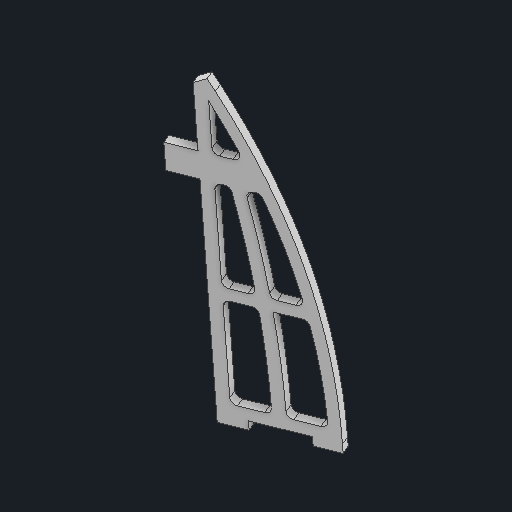
# Autodesk Inventor part: sponson_spanner_bottom
Saved by Autodesk Inventor 2023 (Build 270158030, 158C)
## iProperties
Created: 2022-03-22
Part Number: sponson_spanner_bottom
Material: Generic
Document SubType Name: Modeling
Designer: kardo
Density: 1 g/cm^3
Appearance: Default
Mass: 4.88193 g
Surface Area: 52.3251 cm^2
Volume: 4.88193 cm^3
Author: kardo
Autodesk Inventor part; units mm, degrees
ref_plane "YZ Plane" through (0, 0, 0) normal (1, 0, 0) x (0, 1, 0)
ref_plane "XZ Plane" through (0, 0, 0) normal (0, 1, 0) x (-1, 0, 0)
ref_plane "XY Plane" through (0, 0, 0) normal (0, 0, 1) x (1, 0, 0)
derived "parameters_frame.ipt"
derived "stencil_frame.ipt"
sketch "sk_joint_locations" plane through (81.12, 0, 0) normal (1, 0, 0) x (0, 1, 0)
  line L0 (0, 0) -> (122.4, 9.6331) construction
  line L1 (36.465, 28.832) -> (112.2, 28.832) construction
  arc A0 (36.465, 28.832) -> (11.22, 28.376) centre (36.465, -670.197) ccw construction
  line L2 (-241.5001, 19.2432) -> (11.22, 28.376) construction
  line L3 (-345, 16.32) -> (-262.2001, 18.586) construction
  arc A1 (-262.2001, 18.586) -> (-241.5001, 19.2432) centre (-326.8578, 2381.2399) ccw construction
  line L4 (-122.4795, 3121.122) -> (270.8781, -1876.9598) construction
  line L5 (-230.0001, 3089.1136) -> (-230.0001, -1866.0023) construction
  line L6 (-114.9999, 3089.1136) -> (-114.9999, -1866.0023) construction
  line L7 (-345, 3089.1136) -> (-345, -1866.0023) construction
  line L8 (0, 3089.1136) -> (0, -1866.0023) construction
  line L9 (529.622, 47.2379) -> (-602.608, 2.7525) construction
  line L10 (-673.1615, -36.5999) -> (647.9226, 67.3717) construction
  line L11 (189.4528, 29.5173) -> (189.1111, 38.2146) construction
  line L12 (201.105, 36.5853) -> (201.7901, 27.8813) construction
  line L13 (0, 14.144) -> (121.9006, 15.9783) construction
  line L14 (-230.0001, 45.8224) -> (-230.0001, 19.6588) construction
  line L15 (-345, 37.3935) -> (-345, 16.32) construction
  line L16 (-114.9999, 50.9907) -> (-114.9999, 23.8147) construction
  line L17 (0, 52.89) -> (0, 27.9705) construction
  line L18 (119.1768, 50.5875) -> (119.7216, 43.6656) construction
  line L19 (120.2663, 36.7438) -> (119.7216, 43.6656) construction
  line L20 (120.2663, 36.7438) -> (120.8111, 29.822) construction
  line L21 (120.8111, 29.822) -> (121.3559, 22.9001) construction
  line L22 (121.3559, 22.9001) -> (121.9006, 15.9783) construction
  line L23 (0, 14.144) -> (0, 0) construction
  line L24 (112.2, 37.536) -> (112.2, 28.832) construction
  line L25 (112.2, 35.848) -> (112.2, 30.52) construction
  spline S0 degree 4 poles (-345, 37.3935) (-258.8686, 45.1235) (-172.5923, 49.7074) (-86.3167, 52.89) (0, 52.89) knots 0 0 0 0 0 1 1 1 1 1
  spline S1 degree 3 poles (0, 52.89) (92.8353, 52.89) (195.0311, 49.5089) (255, 36.448) knots 0 0 0 0 1 1 1 1
  spline S2 degree 2 poles (122.4, 9.6331) (190.08, 14.9596) (255, 36.448) knots 0 0 0 1 1 1
  point P0 (-122.4795, 3121.122)
  point P1 (270.8781, -1876.9598)
  point P2 (189.282, 33.8659)
  point P3 (201.4475, 32.2333)
  point P4 (134.9575, 11.3411)
  point P5 (-345, 26.8568)
  point P6 (-230.0001, 32.7406)
  point P7 (-114.9999, 37.4027)
  point P8 (0, 40.4303)
  point P9 (112.2, 33.184)
sketch "sk_spanner_joints_locations" plane through (0, 122.4, 9.6331) normal (0, 0.9969173, 0.0784591) x (-1, 0, 0)
  line L0 (328.7115, -3.4565) -> (-466.2934, 45.1587) construction
  line L1 (-867.9776, -269.6459) -> (1175.5999, 473.0692) construction
  line L2 (-94.4551, 22.4205) -> (-92.9508, 12.0288) construction
  line L3 (-94.4551, 22.4205) -> (-68.6928, 20.8451) construction
  line L4 (-92.9508, 12.0288) -> (-68.6928, 20.8451) construction
  point P0 (0, 0)
  point P1 (-126.048, 0)
  point P2 (-156, 26.184)
  point P3 (-143.691, 25.4313)
  point P4 (-106.7641, 23.1732)
  point P5 (-101.2251, 9.0216)
  point P6 (-117.7737, 3.0072)
ref_plane "plane_strnger_outer" through (84.12, 0, 0) normal (1, 0, 0) x (0, 1, 0)
sketch "sk_corner_offset" plane through (0, 122.4, 9.6331) normal (0, 0.9969173, 0.0784591) x (-1, 0, 0)
  line L0 (-156, 26.184) -> (-126.048, 0) construction
  line L1 (-126.048, 0) -> (-81.12, 0) construction
  point P0 (0, 0)
  point P1 (-125.7476, 0.8)
  dimension "d7" = 0.8
  dimension "d8" = 0.8
  constraints: 4 end point, 1 horizontal
  measures "d7" distance from line of L0 point (-125.748, 0.8)
  measures "d8" distance from line of point (-125.748, 0.8) L1
sketch "sk_tip_offset" plane through (81.12, 0, 0) normal (1, 0, 0) x (0, 1, 0)
  spline S0 degree 3 poles (0, 52.89) (92.8353, 52.89) (195.0311, 49.5089) (255, 36.448) knots 0 0 0 0 1 1 1 1 construction
  spline S1 degree 2 poles (122.4, 9.6331) (190.08, 14.9596) (255, 36.448) knots 0 0 0 1 1 1 construction
  spline S2 degree 5 poles (0, 52.09) (14.1126, 52.09) (28.2252, 52.0249) (42.3374, 51.8877) (70.3021, 51.4557) (98.2587, 50.655) (112.105, 50.1551) (138.5853, 48.9703) (165.0353, 47.2425) (177.6496, 46.2711) (200.1482, 44.2213) (222.5619, 41.3963) (232.3977, 39.9657) (242.2024, 38.3071) (251.9318, 36.2831) knots 0 0 0 0 0 0 0.279151 0.279151 0.279151 0.553204 0.553204 0.553204 0.803431 0.803431 0.803431 1 1 1 1 1 1
  spline S3 degree 4 poles (122.3372, 10.4306) (155.3484, 13.0285) (188.1618, 18.2132) (220.4424, 26.04) (251.9318, 36.2832) knots 0 0 0 0 0 1 1 1 1 1
  point P0 (0, 0)
  dimension "d9" = 0.8
  dimension "d10" = 0.8
  constraints: 1 coincident, 6 other
sketch "sk_spanner_bottom_base" plane through (126.048, 0, 0) normal (0.341579, -0.07374, 0.9369558) x (-0.1718217, 0.9752166, 0.139391)
  spline S0 degree 2 poles (120.7093, -22.4461) (192.8116, -35.8536) (261.4804, 0) knots 0 0 0 1 1 1 construction
  line L0 (-554.724, 148.5277) -> (631.772, -72.103) projected
  line L1 (120.8108, -21.8999) -> (117.8614, -21.3514)
  line L2 (117.8614, -21.3514) -> (119.3693, -13.2422)
  line L3 (119.3693, -13.2422) -> (122.3188, -13.7906)
  line L4 (122.3188, -13.7906) -> (125.5378, 3.5203)
  line L5 (125.5378, 3.5203) -> (122.5883, 4.0688)
  line L6 (122.5883, 4.0688) -> (124.1978, 12.7242)
  line L7 (124.1978, 12.7242) -> (127.1473, 12.1758)
  line L8 (127.1473, 12.1758) -> (128.865, 21.4133)
  line L9 (120.7093, -22.4461) -> (0, 0) construction
  spline S1 degree 2 poles (120.8108, -21.8999) (191.4041, -35.0268) (258.4652, 0.5872) knots 0 0 0 1 1 1
  point P0 (21.6578, 116.4701)
  point P1 (120.7093, -22.4461)
  point P2 (208.6676, 9.8206)
  point P3 (256.8119, -2.3786)
  point P4 (0, 0)
  point P5 (253.8154, -1.8214)
  dimension "d4" = 3
  constraints: 16 end point, 3 parallel, 2 collinear, 2 perpendicular, 1 point on line, 5 other
  measures "d4" distance between parallel lines of L6 L4
extrude "thicken" add sketch "sk_spanner_bottom_base" along normal blind 3
sketch "sk_cut_weight" plane through (126.048, 0, 0) normal (0.341579, -0.07374, 0.9369558) x (-0.1718217, 0.9752166, 0.139391)
  spline S0 degree 2 poles (120.8108, -21.8999) (191.4041, -35.0268) (258.4652, 0.5872) knots 0 0 0 1 1 1 projected
  line L0 (-554.724, 148.5277) -> (631.772, -72.103) projected
  line L1 (122.3188, -13.7906) -> (125.5378, 3.5203) construction
  line L2 (127.1473, 12.1758) -> (128.865, 21.4133) projected
  line L3 (208.6676, 9.8206) -> (203.051, -20.3841) construction
  line L4 (127.1473, 12.1758) -> (200.4675, -1.4582)
  line L5 (200.4675, -1.4582) -> (202.1852, 7.7793)
  line L6 (211.0335, 6.134) -> (209.3158, -3.1036)
  line L7 (209.3158, -3.1036) -> (252.0977, -11.059)
  line L8 (130.3486, 7.5119) -> (199.7362, -5.3908)
  line L9 (130.3486, 7.5119) -> (128.2447, -3.8024)
  line L10 (208.5845, -7.0362) -> (206.9683, -15.7278)
  line L11 (252.0977, -11.059) -> (253.8154, -1.8214)
  line L12 (208.5845, -7.0362) -> (225.3081, -10.146)
  line L13 (165.0424, 1.0605) -> (163.281, -8.412) construction
  line L14 (230.7067, -7.0813) -> (245.2082, -48.1092)
  line L15 (228.4963, -12.8305) -> (226.1658, -6.2369)
  line L16 (252.0977, -11.059) -> (245.2082, -48.1092)
  line L17 (199.7362, -5.3908) -> (198.9374, -9.6866)
  line L18 (128.2447, -3.8024) -> (127.5134, -7.735) construction
  line L19 (198.9374, -9.6866) -> (198.2061, -13.6192) construction
  line L20 (198.2061, -13.6192) -> (197.4073, -17.9149)
  line L21 (163.281, -8.412) -> (162.5497, -12.3445) construction
  line L22 (127.5134, -7.735) -> (125.4095, -19.0494)
  line L23 (162.5497, -12.3445) -> (160.7883, -21.817) construction
  spline S1 degree 2 poles (127.5134, -7.735) (162.4093, -14.0261) (198.2061, -13.6192) knots 0 0 0 1 1 1
  spline S2 degree 2 poles (198.9374, -9.6866) (163.1406, -10.0935) (128.2447, -3.8024) knots 0 0 0 1 1 1
  line L24 (163.0761, 1.4262) -> (161.2788, -8.2394)
  line L25 (160.5475, -12.172) -> (158.7517, -21.8295)
  line L26 (162.8288, -21.7832) -> (164.5539, -12.5064)
  line L27 (165.2852, -8.5738) -> (167.0087, 0.6949)
  spline S3 degree 5 poles (125.4095, -19.0493) (138.1977, -21.1796) (151.1487, -22.3307) (164.1775, -22.4073) (184.4621, -20.7898) (204.3249, -16.5877) (211.4147, -14.7445) (218.413, -12.5908) (225.3081, -10.146) knots 0 0 0 0 0 0 0.639269 0.639269 0.639269 1 1 1 1 1 1
  point P0 (21.6578, 116.4701)
  point P1 (139.2857, 19.818)
  point P2 (232.2417, -11.424)
  dimension "d11" = 3.6057
  dimension "d12" = 3
  dimension "d13" = 6
  dimension "d14" = 4
  dimension "d22" = 60
  dimension "d23" = 4
  dimension "d24" = 4
  dimension "d25" = 4
  dimension "d26" = 4
  dimension "d27" = 4
  constraints: 50 end point, 11 parallel, 7 collinear, 7 perpendicular, 6 point on line, 5 equal length, 2 midpoint, 25 other
  measures "d12" distance between parallel lines of L6 L3
  measures "d13" distance between parallel lines of L3 L5
  measures "d14" distance between parallel lines of L4 L8
  measures "d22" angle of L7 L14
  measures "d23" distance between parallel lines of L15 L14
  measures "d24" distance between parallel lines of L1 L9
  measures "d25" distance of L9.end L18.end
  measures "d26" distance between parallel lines of L26 L25
  measures "d27" distance between parallel lines of L27 L24
extrude "cut_weight" cut sketch "sk_cut_weight" along normal through all both and the other way through all contours L14 L7 S0 | S0 L7 L16 L14 | L7 L6 L0 S0 | S0 L11 L7 | L0 L5 L4 L2 | L8 L24 S2 L9 | L8 L17 S2 L27 | L12 S3 L10 | L20 S3 L26 S1 | L25 S3 L22 S1
extrude "cut_weight_tip" cut sketch "sk_cut_weight" along normal through all both and the other way through all contours L15 L7 L14 S0
extrude "tip_restore" add sketch "sk_cut_weight" along normal blind 3 contours L15 L7 L14 S0
fillet "rounding" radius 2 17 edges at (97.2226, 204.7722, 28.2255) (97.2226, 125.4405, 21.982) (97.2226, 195.8, 27.5194) (105.5315, 205.0092, 25.2151) (122.6141, 126.1645, 12.7822) (119.4541, 159.2603, 16.5389) (109.1951, 196.1414, 23.1815) (109.8425, 162.9739, 20.3352) (111.7981, 125.8561, 16.701) (97.2226, 162.6141, 24.9076) (106.4625, 158.8899, 21.246) (108.0387, 125.7489, 18.0631) (118.7108, 163.2268, 17.122) (106.0831, 162.8667, 21.6973) (97.2226, 158.6264, 24.5938) (105.0886, 196.0243, 24.6694) (101.3291, 195.9171, 26.0315)
equation "\"d7\" = shell_thickness"
equation "\"d8\" = shell_thickness"
equation "\"d9\" = shell_thickness"
equation "\"d10\" = shell_thickness"
equation "\"d4\" = bulkhead_thickness"
equation "\"d5\" = bulkhead_thickness"
equation "\"d12\" = bulkhead_thickness"
equation "\"d13\" = 2 * bulkhead_thickness"
equation "\"d14\" = bulkhead_inset"
equation "\"d23\" = bulkhead_inset"
equation "\"d21\" = 0.5 * bulkhead_inset"
equation "\"d3\" = stringer_thickness"
equation "\"shell_thickness\" = 0.8"
equation "\"bulkhead_thickness\" = 3"
equation "\"bulkhead_inset\" = 4"
equation "\"stringer_thickness\" = 3"
body "Solid1"
